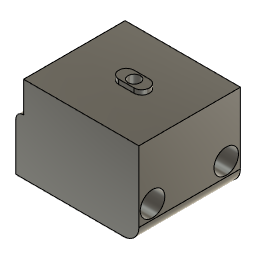
drox-block v1 (Autodesk Fusion 360 design; units mm, degrees)
Autodesk Fusion 360 part; units mm, degrees
sketch "Sketch1" plane through (0, 0, 0) normal (0, 0, 1) x (1, 0, 0)
  line L0 (0, 0) -> (40, 0)
  line L1 (40, 0) -> (40, 33)
  line L2 (40, 33) -> (0, 33)
  line L3 (0, 33) -> (0, 0)
  line L4 (0, 16.5) -> (40, 16.5) construction
  line L5 (2.5, 33) -> (2.5, 0) construction
  line L6 (1.25, 33) -> (1.25, 0) construction
  line L7 (2.5735, 7.5) -> (-0.0735, 7.5)
  line L8 (-0.0735, 7.5) -> (-0.0735, 25.5)
  line L9 (-0.0735, 25.5) -> (2.5735, 25.5)
  line L10 (2.5735, 25.5) -> (2.5735, 7.5)
  line L11 (2.5735, 7.5) -> (-0.0735, 25.5) construction
  line L12 (-0.0735, 7.5) -> (2.5735, 25.5) construction
  line L13 (0, 28.5) -> (40, 28.5) construction
  line L14 (0, 4.5) -> (40, 4.5) construction
  point P0 (1.25, 16.5)
  dimension "d1" = 40
  dimension "d2" = 33
  dimension "d3" = 2.5
  dimension "d4" = 1.25
  dimension "d5" = 18
  dimension "d6" = 24
  dimension "d7" = 12
  constraint horizontal L0
  constraint vertical L1
  constraint horizontal L2
  constraint vertical L3
  constraint coincident L0.start L3.end
  constraint midpoint L3 L4.start
  constraint midpoint L1 L4.end
  constraint coincident L2 L5.start
  constraint perpendicular L2 L5
  constraint coincident L0 L5.end
  constraint coincident L2 L6.start
  constraint coincident L0 L6.end
  constraint perpendicular L0 L6
  constraint horizontal L7
  constraint perpendicular L7 L8
  constraint parallel L7 L9
  constraint parallel L8 L10
  constraint coincident L11 P0
  constraint coincident L12 P0
  constraint midpoint L6 P0
  constraint coincident L3 L13.start
  constraint coincident L1 L13.end
  constraint perpendicular L1 L13
  constraint coincident L3 L14.start
  constraint perpendicular L3 L14
  constraint coincident L1 L14.end
  measures "d1" distance of L0.start L0.end
  measures "d2" distance of L0.start L2.end
  measures "d3" distance of L3 L5
  measures "d4" distance of L3 L6
  measures "d5" distance of L7.end L8.end
  measures "d6" distance of L13 L14
  measures "d7" distance of L4 L13
extrude "Extrude1" add sketch "Sketch1" along normal blind 18 contours L0 L1 L2 L3 L7 L9 L10
extrude "Extrude2" add sketch "Sketch1" along normal blind 11 contours L3 L7 L8 L9 | L3 L7 L9 L10
sketch "Sketch2" plane through (-0.0735, 0, 0) normal (-1, 0, 0) x (0, -1, 0)
  line L0 (-7.5, 0) -> (0, 0)
  line L1 (0, 0) -> (0, 18)
  line L2 (0, 18) -> (-7.5, 18)
  line L3 (-7.5, 18) -> (-7.5, 11)
  line L4 (-25.5, 11) -> (-25.5, 18)
  line L5 (-25.5, 18) -> (-33, 18)
  line L6 (-33, 18) -> (-33, 0)
  line L7 (-28.3891, 0) -> (-28.3891, 18) construction
  line L8 (-4.4379, 0) -> (-4.4379, 18) construction
  line L9 (-33, 9.5) -> (0, 9.5) construction
  circle A0 centre (-4.4379, 9.5) radius 2.05
  circle A1 centre (-28.3891, 9.5) radius 2.1
  circle A2 centre (-4.4379, 9.5) radius 4
  circle A3 centre (-28.3891, 9.5) radius 4
  line L10 (-25.5, 11) -> (-7.5, 11)
  line L11 (-7.5, 11) -> (-7.5, 0)
  line L12 (-33, 0) -> (-25.5, 0)
  line L13 (-25.5, 0) -> (-25.5, 11)
  dimension "d13" = 4.1
  dimension "d14" = 4.2
  dimension "d15" = 8
  dimension "d16" = 8
  dimension "d46" = 1.5
  constraint coincident L0 L7.start
  constraint perpendicular L0 L7
  constraint coincident L5 L7.end
  constraint coincident L0 L8.start
  constraint perpendicular L0 L8
  constraint coincident L2 L8.end
  constraint coincident L6 L9.start
  constraint perpendicular L6 L9
  constraint coincident L1 L9.end
  constraint coincident L8 A0.centre
  constraint coincident L9 A0.centre
  constraint coincident L7 A1.centre
  constraint coincident L9 A1.centre
  constraint concentric A0 A2
  constraint concentric A1 A3
  measures "d13" diameter of A0
  measures "d14" diameter of A1
  measures "d15" diameter of A2
  measures "d16" diameter of A3
  measures "d46" distance of L9 L10
extrude "Extrude3" cut sketch "Sketch2" against normal blind 60 contours A0
extrude "Extrude4" cut sketch "Sketch2" against normal blind 60 contours A1
extrude "Extrude5" cut sketch "Sketch2" against normal blind 60 from surface at -12 contours L3 A2 L11 | A2 L10 L11 | L3 A2 L10
extrude "Extrude6" cut sketch "Sketch2" against normal blind 60 from surface at -12 contours L4 A3 L13 | L4 A3 L10 | A3 L10 L13
sketch "Sketch4" plane through (0, 0, 18) normal (0, 0, 1) x (-1, 0, 0)
  line L0 (-2.5735, -25.5) -> (-2.5735, -7.5)
  line L1 (-2.5735, -7.5) -> (0, -7.5)
  line L2 (0, -7.5) -> (0, 0)
  line L3 (0, 0) -> (-40, 0)
  line L4 (-40, 0) -> (-40, -33)
  line L5 (-40, -33) -> (0, -33)
  line L6 (0, -33) -> (0, -25.5)
  line L7 (0, -25.5) -> (-2.5735, -25.5)
  line L8 (-2.5313, -33) -> (-40, -33)
  line L9 (-40, -33) -> (-40, 0)
  line L10 (-40, 0) -> (-2.5313, 0)
  line L11 (-2.5313, 0) -> (-2.5313, -33)
  constraint horizontal L8
  constraint vertical L9
  constraint horizontal L10
  constraint vertical L11
  constraint coincident L3.end L4.start
  constraint coincident L5 L8.start
extrude "Extrude7" add sketch "Sketch4" along normal blind 10 contours L0 L1 L3 L4 L5 L7 L8 L9 L10 L11 | L0 L1 L7 L11
sketch "Sketch5" plane through (0, 0, 28) normal (0, 0, 1) x (-1, 0, 0)
  line L0 (-2.5313, 0) -> (-40, 0)
  line L1 (-40, 0) -> (-40, -33)
  line L2 (-40, -33) -> (-2.5313, -33)
  line L3 (-2.5313, -33) -> (-2.5313, 0)
  line L4 (-2.5313, -16.5) -> (-40, -16.5) construction
  circle A0 centre (-19.4265, -16.5) radius 2.5
  circle A1 centre (-24.4265, -16.5) radius 2.5
  line L5 (-24.4265, -14) -> (-19.4265, -14)
  line L6 (-19.4265, -14) -> (-19.4265, -19)
  line L7 (-19.4265, -19) -> (-24.4265, -19)
  line L8 (-24.4265, -19) -> (-24.4265, -14)
  line L9 (-24.4265, -14) -> (-19.4265, -19) construction
  line L10 (-19.4265, -14) -> (-24.4265, -19) construction
  line L11 (0.0735, -33) -> (0.0735, 0)
  point P0 (-21.9265, -16.5)
  dimension "d29" = 5
  dimension "d30" = 5
  dimension "d31" = 5
  dimension "d32" = 5
  dimension "d33" = 5
  dimension "d34" = 19.5
  constraint midpoint L3 L4.start
  constraint midpoint L1 L4.end
  constraint coincident L4 A0.centre
  constraint coincident L4 A1.centre
  constraint horizontal L5
  constraint perpendicular L5 L6
  constraint parallel L5 L7
  constraint parallel L6 L8
  constraint coincident L9 P0
  constraint coincident L10 P0
  constraint coincident A0 P0
  constraint coincident L4 P0
  measures "d29" diameter of A0
  measures "d30" diameter of A1
  measures "d31" distance of A0.centre A1.centre
  measures "d32" distance of L6.end L7.end
  measures "d33" distance of L5.end L6.end
  measures "d34" distance of A0.centre L11
extrude "Extrude8" add sketch "Sketch5" along normal blind 1.5 contours A0 L6 | A0 L6 | A0 A1 L5 | A0 A1 L7 | A1 L8 | A1 L8
sketch "Sketch6" plane through (0, 0, 29.5) normal (0, 0, 1) x (-1, 0, 0)
  arc A0 (-24.4265, -14) -> (-24.4265, -19) centre (-24.4265, -16.5) ccw
  line L0 (-24.4265, -19) -> (-19.4265, -19)
  arc A1 (-19.4265, -19) -> (-19.4265, -14) centre (-19.4265, -16.5) ccw
  line L1 (-19.4265, -14) -> (-24.4265, -14)
  circle A2 centre (-21.9753, -16.5) radius 2
  circle A3 centre (-21.9753, -16.5) radius 6
  circle A4 centre (-21.9753, -16.5) radius 2.7
  dimension "d39" = 4
  dimension "d42" = 12
  dimension "d53" = 5.4
  constraint concentric A2 A3
  constraint concentric A2 A4
  measures "d39" diameter of A2
  measures "d42" diameter of A3
  measures "d53" diameter of A4
extrude "Extrude9" cut sketch "Sketch6" against normal blind 58 contours A2
extrude "Extrude10" cut sketch "Sketch6" against normal blind 20 from surface at -15 contours A0 L0 L1 A4 | L1 A4 | L0 L1 A4 | L0 A4 | L0 A1 L1 A4 | A3
fillet "Fillet1" radius 5 1 edges at (40, 16.5, 0)
fillet "Fillet2" radius 2.5 1 edges at (0, 3.75, 18)
fillet "Fillet3" radius 2.5 1 edges at (0, 29.25, 18)
extrude "Extrude11" cut sketch "Sketch6" against normal blind 27 from surface at -8 contours L1 A4 | L0 L1 A4 | L0 A4
equation "d34 = 17 mm + 2.5 mm"
